Autodesk Fusion 360 part; units mm, degrees
note: some values were not read from the file. Set by a fixed rule: which sketch regions a step uses.
(part 4 of 8)
  spline S996 degree 3 poles (60.3742, -134.8859) (60.7619, -135.4599) (60.9507, -136.1616) (61.0041, -136.8621) knots 0 0 0 0 1 1 1 1
  spline S997 degree 3 poles (61.0041, -136.8621) (61.0358, -137.2793) (61.0221, -137.7002) (61.0731, -138.1153) knots 0 0 0 0 1 1 1 1
  spline S998 degree 3 poles (61.0731, -138.1153) (61.1241, -138.5305) (61.2474, -138.9506) (61.5142, -139.2627) knots 0 0 0 0 1 1 1 1
  spline S999 degree 3 poles (61.5142, -139.2627) (61.7586, -139.5486) (62.1056, -139.7213) (62.4621, -139.8115) knots 0 0 0 0 1 1 1 1
  spline S1000 degree 3 poles (62.4621, -139.8115) (62.8185, -139.9016) (63.188, -139.9159) (63.5545, -139.9295) knots 0 0 0 0 1 1 1 1
  spline S1001 degree 3 poles (63.5545, -139.9295) (74.7727, -140.3463) (85.9959, -140.6131) (97.2206, -140.7296) knots 0 0 0 0 1 1 1 1
  spline S1002 degree 3 poles (97.2206, -140.7296) (97.676, -140.6517) (98.1146, -140.4682) (98.4958, -140.1962) knots 0 0 0 0 1 1 1 1
  spline S1003 degree 3 poles (98.4958, -140.1962) (98.8229, -139.9628) (99.1076, -139.6647) (99.3304, -139.3223) knots 0 0 0 0 1 1 1 1
  line L282 (99.3304, -139.3223) -> (99.9372, -136.2235)
  spline S1004 degree 3 poles (99.9372, -136.2235) (100.0613, -135.8344) (100.2795, -135.4786) (100.5658, -135.1984) knots 0 0 0 0 1 1 1 1
  spline S1005 degree 3 poles (100.5658, -135.1984) (101.0219, -134.752) (101.6522, -134.5063) (102.2764, -134.5316) knots 0 0 0 0 1 1 1 1
  line L283 (102.2764, -134.5316) -> (107.1815, -134.4616)
  spline S1006 degree 3 poles (107.1815, -134.4616) (107.9143, -134.5257) (108.6686, -134.2336) (109.1845, -133.6857) knots 0 0 0 0 1 1 1 1
  spline S1007 degree 3 poles (109.1845, -133.6857) (109.5657, -133.2809) (109.8127, -132.7545) (109.9642, -132.209) knots 0 0 0 0 1 1 1 1
  spline S1008 degree 3 poles (109.9642, -132.209) (110.1158, -131.6634) (110.1766, -131.0955) (110.2357, -130.5307) knots 0 0 0 0 1 1 1 1
  line L284 (110.2357, -130.5307) -> (110.9042, -124.136)
  spline S1009 degree 3 poles (110.9042, -124.136) (111.1461, -122.8403) (111.6793, -121.6051) (112.4484, -120.5583) knots 0 0 0 0 1 1 1 1
  spline S1010 degree 3 poles (112.4484, -120.5583) (114.0394, -118.3929) (116.6466, -117.111) (119.2579, -117.1229) knots 0 0 0 0 1 1 1 1
  spline S1011 degree 3 poles (119.2579, -117.1229) (120.024, -117.1262) (120.7895, -117.2342) (121.5292, -117.443) knots 0 0 0 0 1 1 1 1
  line L285 (121.5292, -117.443) -> (121.7392, -119.764)
  spline S1012 degree 3 poles (121.7392, -119.764) (121.7704, -120.173) (121.937, -120.5694) (122.2042, -120.87) knots 0 0 0 0 1 1 1 1
  spline S1013 degree 3 poles (122.2042, -120.87) (122.5163, -121.2211) (122.9512, -121.4328) (123.398, -121.5401) knots 0 0 0 0 1 1 1 1
  spline S1014 degree 3 poles (123.398, -121.5401) (123.8448, -121.6475) (124.3071, -121.6579) (124.7656, -121.6587) knots 0 0 0 0 1 1 1 1
  spline S1015 degree 3 poles (124.7656, -121.6587) (126.6366, -121.662) (128.5108, -121.513) (130.3766, -121.6587) knots 0 0 0 0 1 1 1 1
  spline S1016 degree 3 poles (130.3766, -121.6587) (130.6704, -121.6816) (130.9649, -121.7121) (131.2513, -121.7841) knots 0 0 0 0 1 1 1 1
  spline S1017 degree 3 poles (131.2513, -121.7841) (131.5378, -121.8561) (131.8174, -121.9713) (132.0563, -122.1517) knots 0 0 0 0 1 1 1 1
  spline S1018 degree 3 poles (132.0563, -122.1517) (132.3935, -122.4065) (132.636, -122.7827) (132.7851, -123.1889) knots 0 0 0 0 1 1 1 1
  spline S1019 degree 3 poles (132.7851, -123.1889) (132.9343, -123.5951) (132.9951, -124.0315) (133.0172, -124.466) knots 0 0 0 0 1 1 1 1
  spline S1020 degree 3 poles (133.0172, -124.466) (133.0596, -125.2993) (132.9635, -126.1326) (132.927, -126.9662) knots 0 0 0 0 1 1 1 1
  spline S1021 degree 3 poles (132.927, -126.9662) (132.8987, -127.6134) (132.9059, -128.2665) (132.7862, -128.9022) knots 0 0 0 0 1 1 1 1
  spline S1022 degree 3 poles (132.7862, -128.9022) (132.6666, -129.5379) (132.4046, -130.1686) (131.93, -130.5852) knots 0 0 0 0 1 1 1 1
  spline S1023 degree 3 poles (131.93, -130.5852) (131.4935, -130.9685) (130.9149, -131.137) (130.3459, -131.1734) knots 0 0 0 0 1 1 1 1
  spline S1024 degree 3 poles (130.3459, -131.1734) (129.777, -131.2099) (129.2083, -131.1253) (128.6421, -131.0567) knots 0 0 0 0 1 1 1 1
  spline S1025 degree 3 poles (128.6421, -131.0567) (128.2383, -131.0079) (127.8317, -130.9667) (127.4391, -130.8571) knots 0 0 0 0 1 1 1 1
  spline S1026 degree 3 poles (127.4391, -130.8571) (127.3379, -130.8289) (127.2344, -130.7942) (127.156, -130.7215) knots 0 0 0 0 1 1 1 1
  spline S1027 degree 3 poles (127.156, -130.7215) (127.0808, -130.6519) (127.0345, -130.5494) (127.0307, -130.4445) knots 0 0 0 0 1 1 1 1
  line L286 (127.0307, -130.4445) -> (126.8954, -128.0116)
  spline S1028 degree 3 poles (126.8954, -128.0116) (126.8848, -127.8234) (126.7846, -127.6429) (126.633, -127.5411) knots 0 0 0 0 1 1 1 1
  spline S1029 degree 3 poles (126.633, -127.5411) (126.5291, -127.4714) (126.4034, -127.4382) (126.2803, -127.4479) knots 0 0 0 0 1 1 1 1
  line L287 (126.2803, -127.4479) -> (122.8167, -127.4863)
  spline S1030 degree 3 poles (122.8167, -127.4863) (122.6784, -127.4907) (122.5434, -127.5628) (122.4598, -127.6779) knots 0 0 0 0 1 1 1 1
  spline S1031 degree 3 poles (122.4598, -127.6779) (122.4201, -127.7324) (122.3921, -127.7958) (122.3755, -127.862) knots 0 0 0 0 1 1 1 1
  spline S1032 degree 3 poles (122.3755, -127.862) (122.3589, -127.9283) (122.3544, -127.9971) (122.351, -128.0655) knots 0 0 0 0 1 1 1 1
  line L288 (122.351, -128.0655) -> (121.75, -140.3201)
  spline S1033 degree 3 poles (121.75, -140.3201) (121.8144, -141.4596) (121.4309, -142.6198) (120.7073, -143.4744) knots 0 0 0 0 1 1 1 1
  spline S1034 degree 3 poles (120.7073, -143.4744) (119.9707, -144.3444) (118.8905, -144.8861) (117.7807, -144.9421) knots 0 0 0 0 1 1 1 1
  line L289 (117.7807, -144.9421) -> (108.6375, -145.8918)
  spline S1035 degree 3 poles (108.6375, -145.8918) (108.5326, -145.8841) (108.4255, -145.9217) (108.3457, -145.9932) knots 0 0 0 0 1 1 1 1
  spline S1036 degree 3 poles (108.3457, -145.9932) (108.2894, -146.0437) (108.2495, -146.1105) (108.2133, -146.178) knots 0 0 0 0 1 1 1 1
  line L290 (108.2133, -146.178) -> (108.06, -146.4643)
  line L291 (108.06, -146.4643) -> (45.9486, -145.6008)
  spline S1037 degree 3 poles (45.9486, -145.6008) (44.2815, -145.5776) (42.6105, -145.3903) (41.0139, -144.8882) knots 0 0 0 0 1 1 1 1
  spline S1038 degree 3 poles (41.0139, -144.8882) (39.9899, -144.5662) (38.9904, -144.159) (38.028, -143.6718) knots 0 0 0 0 1 1 1 1
  line L292 (38.028, -143.6718) -> (32.8215, -143.5303)
  spline S1039 degree 3 poles (32.8215, -143.5303) (31.3635, -143.466) (29.9528, -142.6521) (29.1233, -141.3965) knots 0 0 0 0 1 1 1 1
  spline S1040 degree 3 poles (29.1233, -141.3965) (28.7046, -140.7628) (28.43, -140.0256) (28.3285, -139.2627) knots 0 0 0 0 1 1 1 1
  line L293 (28.3285, -139.2627) -> (27.915, -126.1432)
  spline S1041 degree 3 poles (27.915, -126.1432) (27.9507, -125.9289) (27.886, -125.6989) (27.7452, -125.5389) knots 0 0 0 0 1 1 1 1
  spline S1042 degree 3 poles (27.7452, -125.5389) (27.6674, -125.4505) (27.5679, -125.3834) (27.4589, -125.3455) knots 0 0 0 0 1 1 1 1
  spline S1043 degree 3 poles (27.4589, -125.3455) (27.35, -125.3077) (27.2318, -125.2993) (27.119, -125.3214) knots 0 0 0 0 1 1 1 1
  line L294 (27.119, -125.3214) -> (24.3404, -125.5424)
  spline S1044 degree 3 poles (24.3404, -125.5424) (24.2278, -125.5088) (24.1063, -125.5085) (23.9935, -125.5416) knots 0 0 0 0 1 1 1 1
  spline S1045 degree 3 poles (23.9935, -125.5416) (23.8808, -125.5747) (23.7772, -125.641) (23.6977, -125.731) knots 0 0 0 0 1 1 1 1
  spline S1046 degree 3 poles (23.6977, -125.731) (23.5694, -125.8763) (23.5081, -126.0836) (23.5355, -126.2793) knots 0 0 0 0 1 1 1 1
  line L295 (23.5355, -126.2793) -> (23.587, -128.5774)
  spline S1047 degree 3 poles (37.1838, -135.3949) (36.9951, -135.3871) (36.8037, -135.464) (36.6713, -135.6049) knots 0 0 0 0 1 1 1 1
  spline S1048 degree 3 poles (36.6713, -135.6049) (36.5389, -135.7459) (36.4684, -135.949) (36.487, -136.1456) knots 0 0 0 0 1 1 1 1
  spline S1049 degree 3 poles (36.487, -136.1456) (36.5036, -136.3202) (36.5891, -136.4859) (36.7177, -136.5984) knots 0 0 0 0 1 1 1 1
  spline S1050 degree 3 poles (36.7177, -136.5984) (36.8464, -136.7109) (37.0163, -136.7696) (37.1838, -136.7623) knots 0 0 0 0 1 1 1 1
  spline S1051 degree 3 poles (37.1838, -136.7623) (37.3463, -136.7557) (37.5062, -136.6865) (37.6243, -136.5696) knots 0 0 0 0 1 1 1 1
  spline S1052 degree 3 poles (37.6243, -136.5696) (37.7425, -136.4528) (37.8174, -136.2886) (37.8271, -136.1188) knots 0 0 0 0 1 1 1 1
  spline S1053 degree 3 poles (37.8271, -136.1188) (37.8375, -135.9357) (37.7714, -135.7499) (37.6512, -135.6162) knots 0 0 0 0 1 1 1 1
  spline S1054 degree 3 poles (37.6512, -135.6162) (37.5311, -135.4826) (37.3591, -135.4023) (37.1838, -135.3949) knots 0 0 0 0 1 1 1 1
  spline S1055 degree 3 poles (47.6453, -135.6434) (47.4663, -135.6356) (47.2865, -135.7177) (47.1671, -135.8575) knots 0 0 0 0 1 1 1 1
  spline S1056 degree 3 poles (47.1671, -135.8575) (47.0477, -135.9972) (46.9898, -136.191) (47.0072, -136.3775) knots 0 0 0 0 1 1 1 1
  spline S1057 degree 3 poles (47.0072, -136.3775) (47.0226, -136.542) (47.0958, -136.7006) (47.2122, -136.8125) knots 0 0 0 0 1 1 1 1
  spline S1058 degree 3 poles (47.2122, -136.8125) (47.3286, -136.9243) (47.4874, -136.9875) (47.6453, -136.9806) knots 0 0 0 0 1 1 1 1
  spline S1059 degree 3 poles (47.6453, -136.9806) (47.7991, -136.974) (47.9486, -136.9012) (48.0553, -136.7853) knots 0 0 0 0 1 1 1 1
  spline S1060 degree 3 poles (48.0553, -136.7853) (48.162, -136.6694) (48.2255, -136.512) (48.2344, -136.3513) knots 0 0 0 0 1 1 1 1
  spline S1061 degree 3 poles (48.2344, -136.3513) (48.244, -136.1775) (48.1891, -135.9999) (48.0809, -135.8677) knots 0 0 0 0 1 1 1 1
  spline S1062 degree 3 poles (48.0809, -135.8677) (47.9727, -135.7354) (47.8117, -135.6508) (47.6453, -135.6434) knots 0 0 0 0 1 1 1 1
  spline S1063 degree 3 poles (58.0647, -135.9268) (57.8857, -135.919) (57.7058, -136.0011) (57.5864, -136.1409) knots 0 0 0 0 1 1 1 1
  spline S1064 degree 3 poles (57.5864, -136.1409) (57.4671, -136.2806) (57.4092, -136.4745) (57.4266, -136.661) knots 0 0 0 0 1 1 1 1
  spline S1065 degree 3 poles (57.4266, -136.661) (57.4419, -136.8254) (57.5152, -136.984) (57.6315, -137.0959) knots 0 0 0 0 1 1 1 1
  spline S1066 degree 3 poles (57.6315, -137.0959) (57.7479, -137.2077) (57.9068, -137.2709) (58.0647, -137.264) knots 0 0 0 0 1 1 1 1
  spline S1067 degree 3 poles (58.0647, -137.264) (58.2184, -137.2574) (58.3679, -137.1846) (58.4746, -137.0687) knots 0 0 0 0 1 1 1 1
  spline S1068 degree 3 poles (58.4746, -137.0687) (58.5813, -136.9528) (58.6449, -136.7954) (58.6537, -136.6347) knots 0 0 0 0 1 1 1 1
  spline S1069 degree 3 poles (58.6537, -136.6347) (58.6633, -136.4609) (58.6085, -136.2833) (58.5002, -136.1511) knots 0 0 0 0 1 1 1 1
  spline S1070 degree 3 poles (58.5002, -136.1511) (58.392, -136.0188) (58.231, -135.9342) (58.0647, -135.9268) knots 0 0 0 0 1 1 1 1
  spline S1071 degree 3 poles (102.3789, -136.7603) (102.1999, -136.7526) (102.02, -136.8346) (101.9007, -136.9744) knots 0 0 0 0 1 1 1 1
  spline S1072 degree 3 poles (101.9007, -136.9744) (101.7813, -137.1141) (101.7234, -137.308) (101.7408, -137.4945) knots 0 0 0 0 1 1 1 1
  spline S1073 degree 3 poles (101.7408, -137.4945) (101.7561, -137.659) (101.8294, -137.8176) (101.9457, -137.9294) knots 0 0 0 0 1 1 1 1
  spline S1074 degree 3 poles (101.9457, -137.9294) (102.0621, -138.0412) (102.221, -138.1044) (102.3789, -138.0975) knots 0 0 0 0 1 1 1 1
  spline S1075 degree 3 poles (102.3789, -138.0975) (102.5326, -138.0909) (102.6821, -138.0181) (102.7888, -137.9022) knots 0 0 0 0 1 1 1 1
  spline S1076 degree 3 poles (102.7888, -137.9022) (102.8955, -137.7863) (102.9591, -137.6289) (102.9679, -137.4683) knots 0 0 0 0 1 1 1 1
  spline S1077 degree 3 poles (102.9679, -137.4683) (102.9775, -137.2945) (102.9227, -137.1169) (102.8145, -136.9846) knots 0 0 0 0 1 1 1 1
  spline S1078 degree 3 poles (102.8145, -136.9846) (102.7063, -136.8523) (102.5452, -136.7677) (102.3789, -136.7603) knots 0 0 0 0 1 1 1 1
  spline S1079 degree 3 poles (112.6445, -136.9604) (112.4655, -136.9526) (112.2856, -137.0347) (112.1663, -137.1744) knots 0 0 0 0 1 1 1 1
  spline S1080 degree 3 poles (112.1663, -137.1744) (112.0469, -137.3142) (111.989, -137.508) (112.0064, -137.6945) knots 0 0 0 0 1 1 1 1
  spline S1081 degree 3 poles (112.0064, -137.6945) (112.0217, -137.859) (112.095, -138.0176) (112.2113, -138.1294) knots 0 0 0 0 1 1 1 1
  spline S1082 degree 3 poles (112.2113, -138.1294) (112.3277, -138.2413) (112.4866, -138.3044) (112.6445, -138.2976) knots 0 0 0 0 1 1 1 1
  spline S1083 degree 3 poles (112.6445, -138.2976) (112.7982, -138.291) (112.9477, -138.2182) (113.0544, -138.1023) knots 0 0 0 0 1 1 1 1
  spline S1084 degree 3 poles (113.0544, -138.1023) (113.1611, -137.9864) (113.2247, -137.8289) (113.2335, -137.6683) knots 0 0 0 0 1 1 1 1
  spline S1085 degree 3 poles (113.2335, -137.6683) (113.243, -137.4945) (113.1883, -137.3169) (113.0801, -137.1846) knots 0 0 0 0 1 1 1 1
  spline S1086 degree 3 poles (113.0801, -137.1846) (112.9719, -137.0523) (112.8108, -136.9677) (112.6445, -136.9604) knots 0 0 0 0 1 1 1 1
  spline S1087 degree 2 poles (10.8405, -247.7567) (10.8135, -245.439) (10.8536, -244.1565) knots 0 0 0 1 1 1
  spline S1088 degree 3 poles (10.8536, -244.1565) (10.8583, -244.0029) (11.014, -243.8452) (11.2535, -243.8442) knots 0 0 0 0 1 1 1 1
  spline S1089 degree 3 poles (11.2535, -243.8442) (11.7353, -243.8423) (12.7093, -243.8633) (13.04, -243.8642) knots 0 0 0 0 1 1 1 1
  spline S1090 degree 3 poles (13.04, -243.8642) (13.2801, -243.8652) (13.4091, -243.7189) (13.4111, -243.5834) knots 0 0 0 0 1 1 1 1
  spline S1091 degree 3 poles (13.4675, -238.9885) (13.4703, -238.7696) (13.2942, -238.6) (13.018, -238.5972) knots 0 0 0 0 1 1 1 1
  spline S1092 degree 3 poles (13.018, -238.5972) (11.7216, -238.5841) (11.9339, -238.5924) (11.2664, -238.5895) knots 0 0 0 0 1 1 1 1
  spline S1093 degree 3 poles (11.2664, -238.5895) (11.1383, -238.589) (11.0484, -238.4933) (11.0471, -238.2828) knots 0 0 0 0 1 1 1 1
  spline S1094 degree 3 poles (11.0471, -238.2828) (11.0377, -236.7977) (11.0138, -236.8012) (11.0118, -234.9383) knots 0 0 0 0 1 1 1 1
  spline S1095 degree 3 poles (11.0118, -234.9383) (11.0116, -234.712) (10.9737, -234.6195) (11.22, -234.6222) knots 0 0 0 0 1 1 1 1
  line L296 (11.22, -234.6222) -> (17.234, -234.6876)
  spline S1096 degree 3 poles (17.234, -234.6876) (17.5199, -234.6905) (17.6016, -234.7684) (17.595, -235.029) knots 0 0 0 0 1 1 1 1
  spline S1097 degree 3 poles (17.595, -235.029) (17.5771, -235.7343) (17.8248, -236.2023) (18.8717, -236.2473) knots 0 0 0 0 1 1 1 1
  line L297 (18.8717, -236.2473) -> (20.0673, -236.2531)
  spline S1098 degree 2 poles (20.0673, -236.2531) (20.0975, -238.5747) (20.1138, -239.7773) knots 0 0 0 1 1 1
  spline S1099 degree 3 poles (20.1138, -239.7773) (20.1155, -239.9019) (19.9295, -240.0316) (19.7723, -240.0352) knots 0 0 0 0 1 1 1 1
  spline S1100 degree 3 poles (19.7723, -240.0352) (19.0844, -240.0508) (19.0753, -240.0698) (18.4454, -240.0641) knots 0 0 0 0 1 1 1 1
  spline S1101 degree 3 poles (18.4454, -240.0641) (18.2381, -240.0621) (17.9955, -240.2226) (17.9996, -240.3868) knots 0 0 0 0 1 1 1 1
  spline S1102 degree 3 poles (17.9996, -240.3868) (18.0296, -241.5801) (18.0299, -241.5846) (18.0785, -243.2021) knots 0 0 0 0 1 1 1 1
  spline S1103 degree 3 poles (18.0785, -243.2021) (18.0816, -243.3041) (17.9678, -243.4421) (17.8391, -243.4422) knots 0 0 0 0 1 1 1 1
  spline S1104 degree 3 poles (17.8391, -243.4422) (17.5699, -243.4424) (17.4993, -243.449) (17.2111, -243.4553) knots 0 0 0 0 1 1 1 1
  spline S1105 degree 3 poles (17.2111, -243.4553) (17.0652, -243.4582) (16.9282, -243.585) (16.93, -243.6937) knots 0 0 0 0 1 1 1 1
  line L298 (16.93, -243.6937) -> (16.9954, -247.7723)
  line L299 (16.9954, -247.7723) -> (10.8405, -247.7567)
  spline S1106 degree 2 poles (47.9037, -247.8672) (47.8746, -245.9723) (47.8344, -244.6899) knots 0 0 0 1 1 1
  spline S1107 degree 3 poles (47.8344, -244.6899) (47.8297, -244.5362) (47.674, -244.3785) (47.4345, -244.3776) knots 0 0 0 0 1 1 1 1
  spline S1108 degree 3 poles (47.4345, -244.3776) (46.9528, -244.3756) (45.9787, -244.3966) (45.6481, -244.3976) knots 0 0 0 0 1 1 1 1
  spline S1109 degree 3 poles (45.6481, -244.3976) (45.408, -244.3985) (45.279, -244.2522) (45.277, -244.1167) knots 0 0 0 0 1 1 1 1
  spline S1110 degree 3 poles (45.277, -244.1167) (45.2456, -241.9931) (45.2524, -241.992) (45.2206, -239.5218) knots 0 0 0 0 1 1 1 1
  spline S1111 degree 3 poles (45.2206, -239.5218) (45.2177, -239.303) (45.3938, -239.1333) (45.6701, -239.1305) knots 0 0 0 0 1 1 1 1
  spline S1112 degree 3 poles (45.6701, -239.1305) (46.9664, -239.1174) (46.7542, -239.1257) (47.4216, -239.1228) knots 0 0 0 0 1 1 1 1
  spline S1113 degree 3 poles (47.4216, -239.1228) (47.5497, -239.1223) (47.6396, -239.0267) (47.641, -238.8161) knots 0 0 0 0 1 1 1 1
  spline S1114 degree 3 poles (47.641, -238.8161) (47.6504, -237.3311) (47.6743, -237.3345) (47.6762, -235.4716) knots 0 0 0 0 1 1 1 1
  spline S1115 degree 3 poles (47.6762, -235.4716) (47.6765, -235.2453) (47.7144, -235.1528) (47.468, -235.1555) knots 0 0 0 0 1 1 1 1
  line L300 (47.468, -235.1555) -> (41.454, -235.2209)
  spline S1116 degree 3 poles (41.454, -235.2209) (41.1681, -235.2238) (41.1527, -235.2492) (41.1593, -235.5098) knots 0 0 0 0 1 1 1 1
  spline S1117 degree 3 poles (41.1593, -235.5098) (41.1772, -236.2151) (40.9295, -236.6045) (39.8825, -236.6494) knots 0 0 0 0 1 1 1 1
  line L301 (39.8825, -236.6494) -> (38.538, -236.6027)
  spline S1118 degree 2 poles (38.538, -236.6027) (38.5243, -238.6489) (38.508, -239.8515) knots 0 0 0 1 1 1
  spline S1119 degree 3 poles (38.508, -239.8515) (38.5063, -239.9761) (38.6923, -240.1058) (38.8495, -240.1094) knots 0 0 0 0 1 1 1 1
  spline S1120 degree 3 poles (38.8495, -240.1094) (39.5374, -240.125) (39.0166, -240.1309) (39.6465, -240.1251) knots 0 0 0 0 1 1 1 1
  spline S1121 degree 3 poles (39.6465, -240.1251) (39.8538, -240.1232) (40.0911, -240.2836) (40.0923, -240.4479) knots 0 0 0 0 1 1 1 1
  spline S1122 degree 3 poles (40.1127, -243.3681) (40.1135, -243.4701) (40.2234, -243.6081) (40.3522, -243.6082) knots 0 0 0 0 1 1 1 1
  spline S1123 degree 3 poles (40.3522, -243.6082) (40.6214, -243.6084) (40.6919, -243.615) (40.9801, -243.6213) knots 0 0 0 0 1 1 1 1
  spline S1124 degree 3 poles (40.9801, -243.6213) (41.1261, -243.6242) (41.2616, -243.751) (41.2613, -243.8597) knots 0 0 0 0 1 1 1 1
  line L302 (41.2613, -243.8597) -> (41.3017, -247.8696)
  line L303 (41.3017, -247.8696) -> (47.9037, -247.8672)
  spline S1125 degree 3 poles (7.972, -248.7902) (6.132, -246.6023) (6.2367, -236.1578) (8.0837, -233.724) knots 0 0 0 0 1 1 1 1
  spline S1126 degree 3 poles (8.0837, -233.724) (10.5138, -230.5216) (17.2844, -229.2344) (22.0534, -228.4824) knots 0 0 0 0 1 1 1 1
  spline S1127 degree 3 poles (22.0534, -228.4824) (24.6803, -228.0682) (34.3771, -228.1052) (36.3609, -228.4824) knots 0 0 0 0 1 1 1 1
  spline S1128 degree 3 poles (36.3609, -228.4824) (41.2296, -229.4083) (47.3562, -231.0265) (49.7742, -233.0209) knots 0 0 0 0 1 1 1 1
  spline S1129 degree 3 poles (49.7742, -233.0209) (52.8338, -235.5446) (52.4453, -246.8655) (50.3419, -249.3149) knots 0 0 0 0 1 1 1 1
  spline S1130 degree 3 poles (50.3419, -249.3149) (47.5914, -252.5181) (40.6615, -253.0752) (35.461, -254.2994) knots 0 0 0 0 1 1 1 1
  spline S1131 degree 3 poles (35.461, -254.2994) (33.2289, -254.8249) (24.4747, -254.5872) (22.8643, -254.2841) knots 0 0 0 0 1 1 1 1
  spline S1132 degree 3 poles (22.8643, -254.2841) (17.5981, -253.2927) (10.1077, -251.33) (7.972, -248.7902) knots 0 0 0 0 1 1 1 1
  spline S1133 degree 3 poles (29.2071, -234.149) (31.1554, -234.1519) (32.8348, -235.9638) (32.8503, -237.7693) knots 0 0 0 0 1 1 1 1
  spline S1134 degree 3 poles (32.8503, -237.7693) (32.8635, -239.3155) (31.2253, -241.4577) (29.2734, -241.4421) knots 0 0 0 0 1 1 1 1
  spline S1135 degree 3 poles (29.2734, -241.4421) (27.2686, -241.426) (25.6627, -239.1997) (25.6965, -237.6119) knots 0 0 0 0 1 1 1 1
  spline S1136 degree 3 poles (25.6965, -237.6119) (25.7336, -235.8694) (27.3382, -234.1463) (29.2071, -234.149) knots 0 0 0 0 1 1 1 1
  spline S1137 degree 3 poles (29.174, -230.3975) (28.7129, -230.4043) (28.235, -230.8456) (28.2467, -231.2108) knots 0 0 0 0 1 1 1 1
  spline S1138 degree 3 poles (28.2467, -231.2108) (28.2594, -231.6064) (28.8075, -232.0706) (29.3065, -232.0503) knots 0 0 0 0 1 1 1 1
  spline S1139 degree 3 poles (29.3065, -232.0503) (29.7611, -232.0317) (30.1873, -231.571) (30.1676, -231.2108) knots 0 0 0 0 1 1 1 1
  spline S1140 degree 3 poles (30.1676, -231.2108) (30.147, -230.8339) (29.6502, -230.391) (29.174, -230.3975) knots 0 0 0 0 1 1 1 1
  spline S1141 degree 3 poles (29.0747, -243.5146) (28.6136, -243.5213) (28.1356, -243.9626) (28.1473, -244.3278) knots 0 0 0 0 1 1 1 1
  spline S1142 degree 3 poles (28.1473, -244.3278) (28.16, -244.7234) (28.7082, -245.1877) (29.2071, -245.1673) knots 0 0 0 0 1 1 1 1
  spline S1143 degree 3 poles (29.2071, -245.1673) (29.6617, -245.1488) (30.088, -244.688) (30.0682, -244.3278) knots 0 0 0 0 1 1 1 1
  spline S1144 degree 3 poles (30.0682, -244.3278) (30.0476, -243.9509) (29.5508, -243.5081) (29.0747, -243.5146) knots 0 0 0 0 1 1 1 1
  spline S1145 degree 3 poles (22.5833, -236.8249) (22.1222, -236.8316) (21.6442, -237.2729) (21.6559, -237.6381) knots 0 0 0 0 1 1 1 1
  spline S1146 degree 3 poles (21.6559, -237.6381) (21.6686, -238.0337) (22.2168, -238.498) (22.7157, -238.4776) knots 0 0 0 0 1 1 1 1
  spline S1147 degree 3 poles (22.7157, -238.4776) (23.1703, -238.4591) (23.5966, -237.9983) (23.5769, -237.6381) knots 0 0 0 0 1 1 1 1
  spline S1148 degree 3 poles (23.5769, -237.6381) (23.5562, -237.2612) (23.0595, -236.8184) (22.5833, -236.8249) knots 0 0 0 0 1 1 1 1
  spline S1149 degree 3 poles (35.566, -236.9036) (35.1049, -236.9103) (34.627, -237.3517) (34.6387, -237.7168) knots 0 0 0 0 1 1 1 1
  spline S1150 degree 3 poles (34.6387, -237.7168) (34.6514, -238.1124) (35.1996, -238.5767) (35.6985, -238.5563) knots 0 0 0 0 1 1 1 1
  spline S1151 degree 3 poles (35.6985, -238.5563) (36.1531, -238.5378) (36.5793, -238.077) (36.5596, -237.7168) knots 0 0 0 0 1 1 1 1
  spline S1152 degree 3 poles (36.5596, -237.7168) (36.539, -237.3399) (36.0422, -236.8971) (35.566, -236.9036) knots 0 0 0 0 1 1 1 1
  spline S1153 degree 3 poles (18.7911, -250.4272) (18.7541, -249.1872) (18.8052, -248.6019) (18.7746, -247.4497) knots 0 0 0 0 1 1 1 1
  spline S1154 degree 3 poles (18.7746, -247.4497) (18.7676, -247.1897) (18.9433, -246.932) (19.3873, -246.9381) knots 0 0 0 0 1 1 1 1
  spline S1155 degree 3 poles (19.3873, -246.9381) (25.3544, -247.0203) (29.4686, -246.9141) (38.9608, -246.9381) knots 0 0 0 0 1 1 1 1
  spline S1156 degree 3 poles (38.9608, -246.9381) (39.4936, -246.939) (39.8954, -247.0054) (39.9047, -247.3185) knots 0 0 0 0 1 1 1 1
  spline S1157 degree 3 poles (39.9047, -247.3185) (39.9455, -248.6983) (39.9379, -249.1664) (39.9709, -250.9125) knots 0 0 0 0 1 1 1 1
  spline S1158 degree 3 poles (39.9709, -250.9125) (39.9769, -251.226) (39.3725, -251.249) (38.8974, -251.2549) knots 0 0 0 0 1 1 1 1
  spline S1159 degree 3 poles (38.8974, -251.2549) (31.2187, -251.3501) (22.9682, -251.211) (19.6191, -251.2274) knots 0 0 0 0 1 1 1 1
  spline S1160 degree 3 poles (19.6191, -251.2274) (18.9858, -251.261) (18.8054, -250.8879) (18.7911, -250.4272) knots 0 0 0 0 1 1 1 1
  spline S1161 degree 3 poles (31.9139, -197.6636) (20.2225, -197.4099) (12.9497, -204.3308) (13.045, -212.394) knots 0 0 0 0 1 1 1 1
  spline S1162 degree 2 poles (13.045, -212.394) (13.173, -223.2218) (24.1728, -225.9145) knots 0 0 0 1 1 1
  line L304 (24.1728, -225.9145) -> (41.021, -226.1179)
  spline S1163 degree 2 poles (41.021, -226.1179) (51.0689, -223.5461) (50.8874, -212.062) knots 0 0 0 1 1 1
  spline S1164 degree 3 poles (50.8874, -212.062) (50.7886, -205.8081) (43.4439, -197.9452) (31.9139, -197.6636) knots 0 0 0 0 1 1 1 1
  spline S1165 degree 2 poles (17.9976, -215.4524) (18.0401, -217.0521) (18.031, -217.8519) knots 0 0 0 1 1 1
  spline S1166 degree 3 poles (18.031, -217.8519) (18.0271, -218.1975) (18.2075, -218.641) (18.7117, -218.6503) knots 0 0 0 0 1 1 1 1
  spline S1167 degree 2 poles (18.7117, -218.6503) (19.2304, -218.6583) (20.268, -218.6662) knots 0 0 0 1 1 1
  spline S1168 degree 2 poles (20.268, -218.6662) (20.2288, -220.6382) (20.2626, -221.8058) knots 0 0 0 1 1 1
  spline S1169 degree 3 poles (20.2626, -221.8058) (20.2671, -221.9627) (20.4359, -222.1778) (20.6391, -222.1757) knots 0 0 0 0 1 1 1 1
  spline S1170 degree 3 poles (20.6391, -222.1757) (21.9837, -222.1638) (35.1279, -222.1359) (42.3933, -222.1) knots 0 0 0 0 1 1 1 1
  spline S1171 degree 3 poles (42.3933, -222.1) (42.5783, -222.0991) (42.7725, -221.9332) (42.7771, -221.7907) knots 0 0 0 0 1 1 1 1
  spline S1172 degree 3 poles (42.7771, -221.7907) (42.8067, -220.854) (42.7911, -220.4953) (42.789, -219.6936) knots 0 0 0 0 1 1 1 1
  spline S1173 degree 3 poles (42.789, -219.6936) (42.7886, -219.5268) (42.9906, -219.3178) (43.2067, -219.3106) knots 0 0 0 0 1 1 1 1
  spline S1174 degree 2 poles (43.2067, -219.3106) (43.9117, -219.2867) (45.2583, -219.2748) knots 0 0 0 1 1 1
  line L305 (45.2583, -219.2748) -> (45.1995, -216.0039)
  spline S1175 degree 2 poles (45.1995, -216.0039) (43.3125, -215.2321) (43.36, -213.2369) knots 0 0 0 1 1 1
  spline S1176 degree 2 poles (43.36, -213.2369) (43.3954, -211.7494) (45.6177, -210.9023) knots 0 0 0 1 1 1
  line L306 (45.6177, -210.9023) -> (45.6304, -207.8484)
  line L307 (45.6304, -207.8484) -> (43.8522, -207.8285)
  spline S1177 degree 3 poles (43.8522, -207.8285) (43.5994, -207.8257) (43.3172, -207.6079) (43.3182, -207.4129) knots 0 0 0 0 1 1 1 1
  line L308 (43.3182, -207.4129) -> (43.3351, -204.7637)
  spline S1178 degree 3 poles (43.3351, -204.7637) (43.3367, -204.5104) (43.0099, -204.1956) (42.6815, -204.195) knots 0 0 0 0 1 1 1 1
  line L309 (42.6815, -204.195) -> (39.3131, -204.187)
  spline S1179 degree 2 poles (39.3131, -204.187) (39.3189, -204.2029) (39.3362, -203.4102) knots 0 0 0 1 1 1
  spline S1180 degree 3 poles (39.3362, -203.4102) (39.3461, -202.9595) (39.3597, -202.2475) (39.3782, -201.1228) knots 0 0 0 0 1 1 1 1
  spline S1181 degree 3 poles (39.3782, -201.1228) (39.3805, -200.9842) (39.0918, -200.8512) (38.9121, -200.8524) knots 0 0 0 0 1 1 1 1
  spline S1182 degree 3 poles (38.9121, -200.8524) (35.9146, -200.8763) (31.5307, -200.8803) (30.5937, -200.8882) knots 0 0 0 0 1 1 1 1
  spline S1183 degree 3 poles (30.5937, -200.8882) (30.3893, -200.8901) (29.9238, -201.0156) (29.9221, -201.1733) knots 0 0 0 0 1 1 1 1
  spline S1184 degree 3 poles (29.9221, -201.1733) (29.9023, -202.9784) (29.9447, -202.0793) (29.9023, -202.9784) knots 0 0 0 0 1 1 1 1
  spline S1185 degree 3 poles (29.9023, -202.9784) (29.8875, -203.291) (29.3248, -203.6147) (29.0094, -203.6153) knots 0 0 0 0 1 1 1 1
  spline S1186 degree 3 poles (29.0094, -203.6153) (26.7764, -203.619) (23.8143, -203.5953) (21.7901, -203.6073) knots 0 0 0 0 1 1 1 1
  spline S1187 degree 3 poles (21.7901, -203.6073) (21.3934, -203.6101) (21.0876, -203.894) (21.0913, -204.1999) knots 0 0 0 0 1 1 1 1
  spline S1188 degree 3 poles (21.0913, -204.1999) (21.0958, -204.5858) (21.0991, -205.8245) (21.1123, -206.3987) knots 0 0 0 0 1 1 1 1
  spline S1189 degree 3 poles (21.1123, -206.3987) (21.1255, -206.973) (20.7422, -206.8771) (20.4344, -206.8827) knots 0 0 0 0 1 1 1 1
  spline S1190 degree 3 poles (20.4344, -206.8827) (19.7365, -206.8946) (19.2482, -206.9026) (18.9344, -206.9106) knots 0 0 0 0 1 1 1 1
  spline S1191 degree 3 poles (18.9344, -206.9106) (18.6206, -206.9146) (18.5424, -207.0687) (18.5371, -207.2116) knots 0 0 0 0 1 1 1 1
  spline S1192 degree 2 poles (18.5371, -207.2116) (18.505, -208.0774) (18.5482, -209.4297) knots 0 0 0 1 1 1
  spline S1193 degree 3 poles (18.5482, -209.4297) (20.2879, -210.0884) (20.3991, -211.1806) (20.4429, -212.3828) knots 0 0 0 0 1 1 1 1
  spline S1194 degree 3 poles (20.4429, -212.3828) (20.4882, -213.6224) (20.007, -215.1071) (17.9975, -215.4466) knots 0 0 0 0 1 1 1 1
  line L310 (17.9975, -215.4466) -> (17.9976, -215.4524)
  spline S1195 degree 3 poles (18.1865, -212.036) (17.5699, -212.032) (17.2986, -212.4028) (17.3134, -212.7544) knots 0 0 0 0 1 1 1 1
  spline S1196 degree 3 poles (17.3134, -212.7544) (17.3282, -213.1068) (17.6631, -213.384) (18.2221, -213.3797) knots 0 0 0 0 1 1 1 1
  spline S1197 degree 3 poles (18.2221, -213.3797) (18.7207, -213.3759) (19.0488, -213.0357) (19.0482, -212.7332) knots 0 0 0 0 1 1 1 1
  spline S1198 degree 3 poles (19.0482, -212.7332) (19.0474, -212.2948) (18.6113, -212.0395) (18.1865, -212.036) knots 0 0 0 0 1 1 1 1
  spline S1199 degree 3 poles (45.0131, -212.9175) (44.3964, -212.9135) (44.1252, -213.2842) (44.14, -213.6358) knots 0 0 0 0 1 1 1 1
  spline S1200 degree 3 poles (44.14, -213.6358) (44.1548, -213.9882) (44.4897, -214.2653) (45.0487, -214.2611) knots 0 0 0 0 1 1 1 1
  spline S1201 degree 3 poles (45.0487, -214.2611) (45.5473, -214.2573) (45.8754, -213.9174) (45.8748, -213.6146) knots 0 0 0 0 1 1 1 1
  spline S1202 degree 3 poles (45.8748, -213.6146) (45.874, -213.1762) (45.4378, -212.9209) (45.0131, -212.9175) knots 0 0 0 0 1 1 1 1
  spline S1203 degree 3 poles (25.5324, -200.6931) (24.5356, -200.6852) (24.097, -201.3109) (24.1211, -201.9034) knots 0 0 0 0 1 1 1 1
  spline S1204 degree 3 poles (24.1211, -201.9034) (24.1449, -202.4974) (24.6863, -202.9642) (25.5899, -202.957) knots 0 0 0 0 1 1 1 1
  spline S1205 degree 3 poles (25.5899, -202.957) (26.3958, -202.949) (26.9261, -202.3777) (26.9252, -201.8679) knots 0 0 0 0 1 1 1 1
  spline S1206 degree 3 poles (26.9252, -201.8679) (26.9239, -201.1293) (26.2189, -200.699) (25.5324, -200.6931) knots 0 0 0 0 1 1 1 1
  spline S1207 degree 3 poles (106.8928, -62.4564) (107.4964, -63.4292) (126.9166, -59.2915) (130.1603, -59.527) knots 0 0 0 0 1 1 1 1
  spline S1208 degree 3 poles (130.1603, -59.527) (134.4042, -59.8351) (139.1236, -60.8131) (144.2128, -60.7186) knots 0 0 0 0 1 1 1 1
  spline S1209 degree 3 poles (144.2128, -60.7186) (145.4697, -60.6934) (146.6569, -58.2361) (146.2187, -58.2361) knots 0 0 0 0 1 1 1 1
  line L311 (146.2187, -58.2361) -> (144.496, -58.1983)
  line L312 (144.496, -58.1983) -> (144.5786, -54.8717)
  line L313 (144.5786, -54.8717) -> (148.956, -54.8843)
  spline S1210 degree 3 poles (148.956, -54.8843) (150.9779, -54.8885) (153.9813, -45.7143) (153.2508, -43.1916) knots 0 0 0 0 1 1 1 1
  spline S1211 degree 2 poles (153.2508, -43.1916) (153.014, -42.3739) (131.9261, -41.501) knots 0 0 0 1 1 1
  line L314 (131.9261, -41.501) -> (132.4026, -27.2726)
  spline S1212 degree 2 poles (132.4026, -27.2726) (152.5474, -28.2072) (153.5693, -27.6017) knots 0 0 0 1 1 1
  spline S1213 degree 3 poles (153.5693, -27.6017) (155.7054, -26.3358) (151.7168, -14.9934) (150.5252, -14.978) knots 0 0 0 0 1 1 1 1
  line L315 (150.5252, -14.978) -> (146.7024, -14.9285)
  line L316 (146.7024, -14.9285) -> (146.6904, -11.4281)
  line L317 (146.6904, -11.4281) -> (148.0237, -11.4154)
  spline S1214 degree 2 poles (148.0237, -11.4154) (149.5788, -11.4028) (145.4987, -8.5853) knots 0 0 0 1 1 1
  spline S1215 degree 2 poles (145.4987, -8.5853) (137.5707, -9.6291) (133.6054, -9.3798) knots 0 0 0 1 1 1
  spline S1216 degree 3 poles (133.6054, -9.3798) (125.1412, -8.8474) (109.1931, -3.6324) (108.5916, -4.514) knots 0 0 0 0 1 1 1 1
  spline S1217 degree 3 poles (108.5916, -4.514) (107.7758, -5.7099) (114.2357, -16.9166) (115.5766, -23.5798) knots 0 0 0 0 1 1 1 1
  spline S1218 degree 2 poles (115.5766, -23.5798) (116.1456, -26.407) (115.9835, -32.2387) knots 0 0 0 1 1 1
  line L318 (115.9835, -32.2387) -> (117.8826, -32.2418)
  line L319 (117.8826, -32.2418) -> (117.9364, -35.9926)
  line L320 (117.9364, -35.9926) -> (116.0789, -36.0476)
  spline S1219 degree 2 poles (116.0789, -36.0476) (116.1574, -41.6718) (115.2934, -44.2347) knots 0 0 0 1 1 1
  spline S1220 degree 3 poles (115.2934, -44.2347) (113.7615, -48.7789) (106.2783, -61.4666) (106.8928, -62.4564) knots 0 0 0 0 1 1 1 1
  spline S1221 degree 3 poles (118.2129, -48.0314) (119.0399, -48.0482) (125.8331, -54.9543) (125.6383, -56.2643) knots 0 0 0 0 1 1 1 1
  spline S1222 degree 3 poles (125.6383, -56.2643) (125.4424, -57.5812) (113.821, -59.0095) (113.1236, -58.0021) knots 0 0 0 0 1 1 1 1
  spline S1223 degree 3 poles (113.1236, -58.0021) (112.5258, -57.1387) (117.2145, -48.0134) (118.2129, -48.0314) knots 0 0 0 0 1 1 1 1
  spline S1224 degree 3 poles (115.2591, -9.4091) (114.8423, -10.0128) (118.367, -19.4939) (119.3289, -19.5087) knots 0 0 0 0 1 1 1 1
  spline S1225 degree 3 poles (119.3289, -19.5087) (120.2079, -19.5213) (127.7807, -13.2006) (127.3758, -11.8377) knots 0 0 0 0 1 1 1 1
  spline S1226 degree 3 poles (127.3758, -11.8377) (127.0595, -10.7732) (115.7277, -8.7303) (115.2591, -9.4091) knots 0 0 0 0 1 1 1 1
  line L321 (13.4675, -238.9885) -> (13.4111, -243.5834)
  line L322 (40.1127, -243.3681) -> (40.0923, -240.4479)
extrude "Extrude1" add sketch "Sketch1" along normal blind 3.5 contours S0 S1 L0 S2 S3 | S46 S47 S48 S49 S50 S51 | S52 S53 S54 S55 | S56 S57 S58 S59 | S60 S61 S62 S63 | S64 S65 S66 S67 | S96 S97 S238 S239 L64 S240 S241 S242 L65 S243 S244 L66 S245 S246 S247 S248 S249 S250 S251 S252 S253 S254 S255 S256 S257 L67 | S96 S97 L66 S245 | S169 S170 S171 S172 S173 S174 S175 S176 | L55 L56 S234 S235 L57 S236 S237 L58 L59 L60 L61 L62 | S342 S343 S344 S345 L97 S346 S347 L98 S348 S349 S350 S351 L99 S352 S353 L100 | S438 S439 L122 S440 S441 S442 S443 S444 S445 S446 S447 S448 S449 S450 S451 S452 S453 S454 S455 S456 S457 S458 S459 S460 S461 S462 S463 S464 S465 S466 S467 S468 S469 S470 S471 S472 S473 S474 S475 S476 S477 S478 S479 S480 S481 S482 S483 S484 S485 S486 | S519 S520 S521 S522 S523 S524 S525 S526 S527 S528 S529 S530 S531 L126 S532 S533 S534 S535 S536 S537 S538 S539 S540 S541 S542 S543 | S669 S670 S671 S672 S673 S674 S675 S676 | S693 S694 L146 S695 S696 S697 S698 S699 L147 S700 S701 S702 | S709 S710 S711 S712 S713 L149 S714 S715 S716 S717 L150 S718 S719 S720 S721 L151 S722 S723 S724 S725 L152 S726 S727 S728 L153 S729 S730 S731 S732 S733 S734 L154 S735 S736 S737 S738 S739 L155 S740 S741 L156 S742 S743 S744 S745 L157 S746 S747 S748 S749 L158 S750 S751 L159 S752 S753 S754 S755 S756 L160 S757 S758 S759 L161 S760 S761 S762 S763 L162 S764 S765 L163 S766 S767 L164 S768 S769 S770 S771 L165 S772 S773 L166 S774 S775 S776 L167 S777 S778 S779 S780 L168 S781 S782 L169 S783 S784 L170 S785 S786 S787 S788 S789 S790 L171 S791 S792 S793 S794 L172 S795 S796 S797 S798 L173 S799 S800 L174 S801 S802 L175 S803 S804 S805 S806 S807 L176 S808 S809 L177 S810 S811 S812 S813 L178 S814 S815 S816 L179 S817 S818 L180 | S923 S924 S925 S926 S927 S928 S929 S930 S931 S932 S933 | S946 S947 S948 S949 S950 S951 S952 S953 S954 S955 S956 S957 S958 S959 S960 S961 S962 S963 S964 S965 S966 | S967 S968 S969 S970 S971 L266 L267 L268 L269 L270 S972 S973 S974 S975 S976 L271 L272 L273 L274 L275 L276 L277 | S977 S978 S979 S980 S981 S982 S983 S984 S985 L278 S986 S987 S988 L279 S989 S990 S991 L280 S992 S993 S994 L281 S995 S996 S997 S998 S999 S1000 S1001 S1002 S1003 L282 S1004 S1005 L283 S1006 S1007 S1008 L284 S1009 S1010 S1011 L285 S1012 S1013 S1014 S1015 S1016 S1017 S1018 S1019 S1020 S1021 S1022 S1023 S1024 S1025 S1026 S1027 L286 S1028 S1029 L287 S1030 S1031 S1032 L288 S1033 S1034 L289 S1035 S1036 L290 L291 S1037 S1038 L292 S1039 S1040 L293 S1041 S1042 S1043 L294 S1044 S1045 S1046 L295 | S1125 S1126 S1127 S1128 S1129 S1130 S1131 S1132 | S1161 S1162 L304 S1163 S1164 | S1207 S1208 S1209 L311 L312 L313 S1210 S1211 L314 S1212 S1213 L315 L316 L317 S1214 S1215 S1216 S1217 S1218 L318 L319 L320 S1219 S1220 makes body 1 at (181.1259, 0, 168.5479) makes body 2 at (44.2737, 0, 33.9738) makes body 3 at (119.0604, 0, 135.1901) makes body 4 at (27.2842, 0, 194.2829) makes body 5 at (29.0684, 0, 223.3967) makes body 6 at (97.98, 0, 124.8902) makes body 7 at (27.4631, 0, 39.484) makes body 8 at (147.7875, 0, 37.9969) makes body 9 at (142.853, 0, 173.176) makes body 10 at (227.9699, 0, 208.3358) makes body 11 at (144.0704, 0, 23.3061) makes body 12 at (83.9518, 0, 80.085) makes body 13 at (12.5211, 0, 82.2808) makes body 14 at (22.5124, 0, 243.7392) makes body 15 at (61.6681, 0, 112.2186) makes body 16 at (85.2183, 0, 39.5868) makes body 17 at (101.9238, 0, 36.7697) makes body 18 at (203.1631, 0, 188.2814)